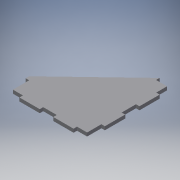
# Autodesk Inventor part: left
Saved by Autodesk Inventor 2016 (Build 200138000, 138)
## iProperties
Created: 2016-05-17
Part Number: left
Material: Generic
Document SubType Name: Modeling
Designer: Lillahunden
Density: 1 g/cm^3
Appearance: Default
Author: Lillahunden
Autodesk Inventor part; units mm, degrees
ref_plane "YZ Plane" through (0, 0, 0) normal (1, 0, 0) x (0, 1, 0)
ref_plane "XZ Plane" through (0, 0, 0) normal (0, 1, 0) x (-1, 0, 0)
ref_plane "XY Plane" through (0, 0, 0) normal (0, 0, 1) x (1, 0, 0)
sketch "Sketch1" plane through (0, 0, 0) normal (0, 0, 1) x (1, 0, 0)
  line L0 (0, 0) -> (23.33, 0) projected
  line L1 (23.33, 0) -> (23.33, 6) projected
  line L2 (0, 6) -> (23.33, 6) projected
  line L3 (0, 0) -> (0, 6) projected
  line L4 (-35.01, 0) -> (0, 0) projected
  line L5 (0, 0) -> (0, 6) projected
  line L6 (-35.01, 6) -> (0, 6) projected
  line L7 (-35.01, 0) -> (-35.01, 6) projected
  line L8 (-58.34, 0) -> (-35.01, 0) projected
  line L9 (-35.01, 0) -> (-35.01, 6) projected
  line L10 (-58.34, 6) -> (-35.01, 6) projected
  line L11 (-58.34, 0) -> (-58.34, 6) projected
  line L12 (-93.34, 0) -> (-58.34, 0) projected
  line L13 (-58.34, 0) -> (-58.34, 6) projected
  line L14 (-93.34, 6) -> (-58.34, 6) projected
  line L15 (-93.34, 0) -> (-93.34, 6) projected
  line L16 (-116.67, 0) -> (-93.34, 0) projected
  line L17 (-93.34, 0) -> (-93.34, 6) projected
  line L18 (-116.67, 6) -> (-93.34, 6) projected
  line L19 (-116.67, 0) -> (-116.67, 6) projected
  line L20 (-110.67, 34) -> (-116.67, 34) projected
  line L21 (-116.67, 6) -> (-116.67, 34) projected
  line L22 (-116.67, 6) -> (-110.67, 6) projected
  line L23 (-110.67, 34) -> (-110.67, 6) projected
  line L24 (23.33, 30.68) -> (17.33, 30.68) projected
  line L25 (17.33, 30.68) -> (17.33, 6) projected
  line L26 (17.33, 6) -> (23.33, 6) projected
  line L27 (23.33, 30.68) -> (23.33, 6) projected
  line L28 (17.33, 30.68) -> (17.33, 65.68) projected
  line L29 (23.33, 30.68) -> (17.33, 30.68) projected
  line L30 (23.33, 65.68) -> (23.33, 30.68) projected
  line L31 (23.33, 65.68) -> (17.33, 65.68) projected
  line L32 (23.33, 90.34) -> (17.33, 90.34) projected
  line L33 (17.33, 90.34) -> (17.33, 65.68) projected
  line L34 (17.33, 65.68) -> (23.33, 65.68) projected
  line L35 (23.33, 90.34) -> (23.33, 65.68) projected
  line L36 (17.33, 90.34) -> (17.33, 125.34) projected
  line L37 (23.33, 90.34) -> (17.33, 90.34) projected
  line L38 (23.33, 125.34) -> (23.33, 90.34) projected
  line L39 (23.33, 125.34) -> (17.33, 125.34) projected
  line L40 (23.33, 144) -> (17.33, 144) projected
  line L41 (17.33, 144) -> (17.33, 125.34) projected
  line L42 (17.33, 125.34) -> (23.33, 125.34) projected
  line L43 (23.33, 144) -> (23.33, 125.34) projected
  line L44 (-1.67, 150) -> (23.33, 150) projected
  line L45 (-1.67, 150) -> (-1.67, 144) projected
  line L46 (23.33, 144) -> (-1.67, 144) projected
  line L47 (23.33, 150) -> (23.33, 144) projected
  line L48 (-110.67, 40) -> (-110.67, 34) projected
  line L49 (-116.67, 40) -> (-110.67, 40) projected
  line L50 (-116.67, 34) -> (-116.67, 40) projected
  line L51 (-116.67, 34) -> (-110.67, 34) projected
  line L52 (-116.67, 40) -> (-1.67, 150)
  constraints: 2 end point
extrude "Extrusion1" add sketch "Sketch1" against normal blind 6 contours L4 L7 L6 L3 | L6 L10 L14 L18 L23 L48 L49 L52 L45 L46 L41 L36 L33 L28 L25 L2 | L12 L15 L14 L11 | L24 L28 L31 L30 | L32 L36 L39 L38 | L20 L50 L49 L48
body "Solid1"
